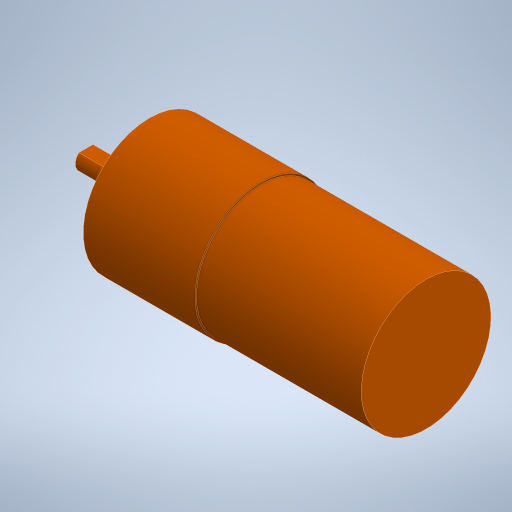
# Autodesk Inventor part: motor6kg
Saved by Autodesk Inventor 2024.3 (Build 283343000, 343)
## iProperties
Created: 2024-05-15
Part Number: motor6kg
Material: Generic
Document SubType Name: Modeling
Designer: USUARIO
Density: 1 g/cm^3
Appearance: Default(1)
Mass: 24.9336 g
Surface Area: 53.0545 cm^2
Volume: 24.9336 cm^3
Author: USUARIO
Autodesk Inventor part; units mm, degrees
ref_plane "YZ Plane" through (0, 0, 0) normal (1, 0, 0) x (0, 1, 0)
ref_plane "XZ Plane" through (0, 0, 0) normal (0, 1, 0) x (-1, 0, 0)
ref_plane "XY Plane" through (0, 0, 0) normal (0, 0, 1) x (1, 0, 0)
sketch "Sketch1" plane through (0, 0, 0) normal (1, 0, 0) x (0, 1, 0)
  circle A0 centre (0, 0) radius 12.2
  circle A1 centre (0, 0) radius 12.5
  dimension "d0" = 24.4
  dimension "d1" = 25
  constraints: 2 centre point, 2 coincident
  measures "d0" diameter of A0
  measures "d1" diameter of A1
extrude "Extrusion1" add sketch "Sketch1" along normal blind 31 contours A0
extrude "Extrusion2" add sketch "Sketch1" against normal blind 21 contours A0 | A1
sketch "Sketch2" plane through (-21, 0, 0) normal (-1, 0, 0) x (0, 0, 1)
  circle A0 centre (0, 0) radius 3.5
  dimension "d6" = 7
  constraints: 1 centre point, 1 coincident
  measures "d6" diameter of A0
extrude "Extrusion3" add sketch "Sketch2" along normal blind 2.5
sketch "Sketch3" plane through (-23.5, 0, 0) normal (-1, 0, 0) x (0, 0, 1)
  circle A0 centre (0, 0) radius 2
  dimension "d9" = 4
  constraints: 1 centre point, 1 coincident
  measures "d9" diameter of A0
extrude "Extrusion4" add sketch "Sketch3" along normal blind 9.5
sketch "Sketch4" plane through (-33, 0, 0) normal (-1, 0, 0) x (0, 0, 1)
  circle A0 centre (0, 0) radius 2
  circle A1 centre (0, 0) radius 2 projected
  line L0 (-1.3229, 1.5) -> (1.3229, 1.5)
  circle A2 centre (0, 0) radius 2 projected
  dimension "d12" = 4
  dimension "d13" = 3.5
  constraints: 3 point on circle, 2 end point, 1 centre point, 1 coincident, 1 horizontal
  measures "d12" diameter of A0
extrude "Extrusion5" cut sketch "Sketch4" against normal blind 8 contours L0 A0 picked at (-0.3089, 1.5908)
sketch "Sketch5" plane through (-21, 0, 0) normal (-1, 0, 0) x (0, 0, 1)
  arc A0 (-1.3229, 1.5) -> (1.3229, 1.5) centre (0, 0) ccw projected
  line L0 (0, 0) -> (0, 8.5) construction
  circle A1 centre (0, 8.5) radius 1.25
  line L1 (0, 0) -> (0, -8.5) construction
  circle A2 centre (0, -8.5) radius 1.25
  dimension "d16" = 8.5
  dimension "d17" = 2.5
  dimension "d18" = 8.5
  dimension "d19" = 2.5
  constraints: 4 end point, 3 coincident, 2 centre point, 2 vertical
  measures "d16" distance of L0.start L0.end
  measures "d17" diameter of A1
  measures "d18" distance of L0.start L1.end
  measures "d19" diameter of A2
extrude "Extrusion6" cut sketch "Sketch5" against normal blind 8
thread "Thread1" size "M3x0.5" class "6H" standard "ANSI Metric M Profile" full length
thread "Thread2" size "M3x0.5" class "6H" standard "ANSI Metric M Profile" full length
body "Solid1"
